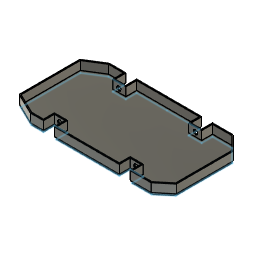
RPi_4_dummy_v5 v7 (Autodesk Fusion 360 design; units mm, degrees)
Autodesk Fusion 360 part; units mm, degrees
sketch "Sketch1" plane through (0, 0, 0) normal (0, 0, 1) x (1, 0, 0)
  line L0 (25.4, -17.78) -> (63.5, -17.78)
  line L1 (63.5, -17.78) -> (63.5, 109.22)
  line L2 (63.5, 109.22) -> (215.9, 109.22)
  line L3 (215.9, 109.22) -> (215.9, -17.78)
  line L4 (215.9, -17.78) -> (952.5, -17.78)
  line L5 (952.5, -17.78) -> (952.5, 109.22)
  line L6 (952.5, 109.22) -> (1104.9, 109.22)
  line L7 (1104.9, 109.22) -> (1104.9, -17.78)
  line L8 (1104.9, -17.78) -> (1333.5, -17.78)
  line L9 (1333.5, -17.78) -> (1485.9, 109.22)
  line L10 (1485.9, 109.22) -> (1485.9, 769.62)
  line L11 (1485.9, 769.62) -> (1333.5, 922.02)
  line L12 (215.9, 795.02) -> (63.5, 795.02)
  line L13 (215.9, 795.02) -> (215.9, 922.02)
  line L14 (63.5, 795.02) -> (63.5, 922.02)
  line L15 (215.9, 922.02) -> (571.5, 922.02)
  line L16 (571.5, 922.02) -> (952.5, 922.02)
  line L17 (952.5, 922.02) -> (952.5, 795.02)
  line L18 (952.5, 795.02) -> (1104.9, 795.02)
  line L19 (1104.9, 795.02) -> (1104.9, 922.02)
  line L20 (1104.9, 922.02) -> (1333.5, 922.02)
  line L21 (63.5, 922.02) -> (-114.3, 922.02)
  line L22 (-114.3, 922.02) -> (-317.5, 795.02)
  line L23 (25.4, -17.78) -> (-76.2, -17.78)
  line L24 (-76.2, -17.78) -> (-317.5, 100.121)
  line L25 (-317.5, 100.121) -> (-317.5, 795.02)
  dimension "d1" = 127
  dimension "d2" = 736.6
  dimension "d3" = 152.4
  dimension "d4" = 152.4
  dimension "d6" = 127
  dimension "d7" = 127
  dimension "d8" = 127
  dimension "d9" = 152.4
  dimension "d10" = 127
  dimension "d11" = 177.8
  constraint horizontal L0
  constraint perpendicular L0 L1
  constraint perpendicular L1 L2
  constraint perpendicular L0 L3
  constraint perpendicular L3 L4
  constraint perpendicular L4 L5
  constraint perpendicular L5 L6
  constraint perpendicular L6 L7
  constraint perpendicular L7 L8
  constraint perpendicular L8 L10
  constraint perpendicular L12 L13
  constraint perpendicular L12 L14
  constraint perpendicular L13 L15
  constraint perpendicular L5 L16
  constraint perpendicular L16 L17
  constraint perpendicular L14 L21
  constraint parallel L0 L23
  constraint perpendicular L21 L25
  measures "d1" distance of L0.end L1.end
  measures "d2" distance of L3.end L4.end
  measures "d3" distance of L5.end L6.end
  measures "d4" distance of L12.start L12.end
  measures "d6" distance of L12.start L13.end
  measures "d7" distance of L12.end L14.end
  measures "d8" distance of L16.end L17.end
  measures "d9" distance of L17.end L18.end
  measures "d10" distance of L18.end L19.end
  measures "d11" distance of L14.end L21.end
sketch "Sketch2" plane through (0, 0, 0) normal (0, 0, 1) x (1, 0, 0)
  line L0 (952.5, -17.78) -> (215.9, -17.78)
  line L1 (215.9, -17.78) -> (215.9, 109.22)
  line L2 (215.9, 109.22) -> (215.9, -17.78)
  line L3 (215.9, -17.78) -> (215.9, 109.22)
  line L4 (215.9, 109.22) -> (63.5, 109.22)
  line L5 (63.5, 109.22) -> (63.5, -17.78)
  line L6 (63.5, -17.78) -> (-76.2, -17.78)
  line L7 (-76.2, -17.78) -> (-317.5, 100.121)
  line L8 (-317.5, 100.121) -> (-317.5, 795.02)
  line L9 (-317.5, 795.02) -> (-114.3, 922.02)
  line L10 (-114.3, 922.02) -> (63.5, 922.02)
  line L11 (63.5, 922.02) -> (63.5, 795.02)
  line L12 (63.5, 795.02) -> (215.9, 795.02)
  line L13 (215.9, 795.02) -> (215.9, 922.02)
  line L14 (215.9, 922.02) -> (952.5, 922.02)
  line L15 (952.5, 922.02) -> (952.5, 795.02)
  line L16 (952.5, 795.02) -> (1104.9, 795.02)
  line L17 (1104.9, 795.02) -> (1104.9, 922.02)
  line L18 (1104.9, 922.02) -> (1333.5, 922.02)
  line L19 (1333.5, 922.02) -> (1485.9, 769.62)
  line L20 (1485.9, 769.62) -> (1485.9, 109.22)
  line L21 (1485.9, 109.22) -> (1333.5, -17.78)
  line L22 (1333.5, -17.78) -> (1104.9, -17.78)
  line L23 (1104.9, -17.78) -> (1104.9, 109.22)
  line L24 (1104.9, 109.22) -> (952.5, 109.22)
  line L25 (952.5, 109.22) -> (952.5, -17.78)
  point P0 (952.5, -17.78)
  point P1 (215.9, -17.78)
  point P2 (215.9, 109.22)
  point P3 (63.5, 109.22)
  point P4 (63.5, -17.78)
  point P5 (-76.2, -17.78)
  point P6 (-317.5, 100.121)
  point P7 (-317.5, 795.02)
  point P8 (-114.3, 922.02)
  point P9 (63.5, 922.02)
  point P10 (63.5, 795.02)
  point P11 (215.9, 795.02)
  point P12 (215.9, 922.02)
  point P13 (952.5, 922.02)
  point P14 (952.5, 795.02)
  point P15 (1104.9, 795.02)
  point P16 (1104.9, 922.02)
  point P17 (1333.5, 922.02)
  point P18 (1485.9, 769.62)
  point P19 (1485.9, 109.22)
  point P20 (1333.5, -17.78)
  point P21 (1104.9, -17.78)
  point P22 (1104.9, 109.22)
  point P23 (952.5, 109.22)
  constraint coincident P0 L0.start
  constraint coincident P1 L0.end
  constraint coincident P2 L1.end
  constraint coincident P3 L4.end
  constraint coincident P4 L5.end
  constraint coincident P5 L6.end
  constraint coincident P6 L7.end
  constraint coincident P7 L8.end
  constraint coincident P8 L9.end
  constraint coincident P9 L10.end
  constraint coincident P10 L11.end
  constraint coincident P11 L12.end
  constraint coincident P12 L13.end
  constraint coincident P13 L14.end
  constraint coincident P14 L15.end
  constraint coincident P15 L16.end
  constraint coincident P16 L17.end
  constraint coincident P17 L18.end
  constraint coincident P18 L19.end
  constraint coincident P19 L20.end
  constraint coincident P20 L21.end
  constraint coincident P21 L22.end
  constraint coincident P22 L23.end
  constraint coincident P23 L24.end
extrude "Extrude1" add sketch "Sketch2" along normal blind 25.4 in component "Component"
extrude "Extrude2" add 1 faces at (461.4333, 566.42, 25.4) along direction (0, 0, 1) blind 101.6 thin wall 12.7 outside in component "Component"
hole "Hole1" at (139.7, 96.52, 76.2) direction (0, 1, 0) diameter 50.8 depth 50.8 tip angle 118 in component "Component"
hole "Hole2" at (1031.8357, 807.72, 73.8534) direction (0, -1, 0) diameter 50.8 depth 50.8 tip angle 118 in component "Component"
hole "Hole3" at (133.4205, 807.72, 68.6555) direction (0, -1, 0) diameter 50.8 depth 50.8 tip angle 118 in component "Component"
hole "Hole4" at (1033.0789, 96.52, 75.4731) direction (0, 1, 0) diameter 50.8 depth 50.8 tip angle 118 in component "Component"
component "Component" placed x (1, 0, 0) y (0, 1, 0) z (0, 0, 1) at (0, 0, 0)
